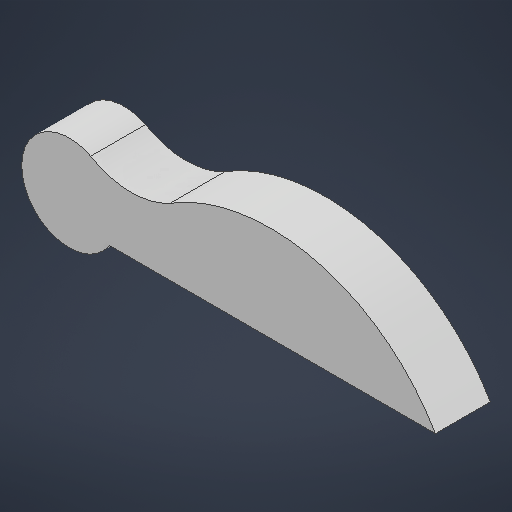
# Autodesk Inventor part: хрень
Saved by Autodesk Inventor 2025 (Build 290162000, 162)
## iProperties
Created: 2024-11-13
Part Number: хрень
Material: Типовые
Document SubType Name: Modeling
Designer: Phantom
Density: 1 g/cm^3
Appearance: По умолчанию
Author: Phantom
Autodesk Inventor part; units mm, degrees
ref_plane "YZ Plane" through (0, 0, 0) normal (1, 0, 0) x (0, 1, 0)
ref_plane "XZ Plane" through (0, 0, 0) normal (0, 1, 0) x (-1, 0, 0)
ref_plane "XY Plane" through (0, 0, 0) normal (0, 0, 1) x (1, 0, 0)
sketch "Эскиз1" plane through (0, 0, 0) normal (0, 0, 1) x (1, 0, 0)
  circle A0 centre (0, 0) radius 13
  arc A1 (5.8567, 11.606) -> (27.5924, 11.3427) centre (16.954, 30.4151) ccw
  line L0 (100.0896, -6.9459) -> (10.9888, -6.9459)
  arc A2 (100.0896, -6.9459) -> (27.5924, 11.3427) centre (55, -32.8481) ccw
  dimension "d0" = 26
  constraints: 6 point on circle, 3 centre point, 2 end point, 1 coincident
  measures "d0" diameter of A0
extrude "Выдавливание1" add sketch "Эскиз1" along normal blind 15 contours A1 A0 | A0 A1 A2 L0 picked at (-2.6021, -3.4241)
